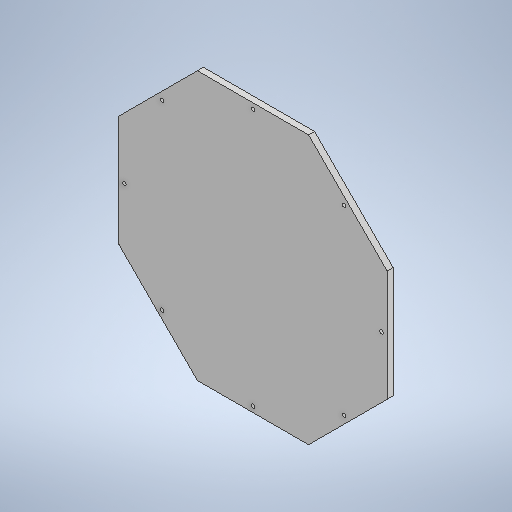
# Autodesk Inventor part: Cap
Saved by Autodesk Inventor 2025.1 (Build 291241020, 241B)
## iProperties
Created: 2024-09-21
Part Number: Cap
Material: 일반
Document SubType Name: Modeling
Designer: daare
Density: 1 g/cm^3
Appearance: 기본값
Author: daare
Autodesk Inventor part; units mm, degrees
ref_plane "YZ Plane" through (0, 0, 0) normal (1, 0, 0) x (0, 1, 0)
ref_plane "XZ Plane" through (0, 0, 0) normal (0, 1, 0) x (-1, 0, 0)
ref_plane "XY Plane" through (0, 0, 0) normal (0, 0, 1) x (1, 0, 0)
sketch "스케치1" plane through (0, 0, 0) normal (0, 0, 1) x (1, 0, 0)
  line L0 (112, -46.3919) -> (46.3919, -112)
  line L1 (46.3919, -112) -> (-46.3919, -112)
  line L2 (-46.3919, -112) -> (-112, -46.3919)
  line L3 (-112, -46.3919) -> (-112, 46.3919)
  line L4 (-112, 46.3919) -> (-46.3919, 112)
  line L5 (-46.3919, 112) -> (46.3919, 112)
  line L6 (46.3919, 112) -> (112, 46.3919)
  line L7 (112, 46.3919) -> (112, -46.3919)
  line L8 (0, 0) -> (-9.429, 0)
  line L9 (0, 0) -> (-9.429, 0)
  circle A0 centre (0, 107.302) radius 1.5
  circle A1 centre (-75.874, 75.874) radius 1.5
  circle A2 centre (-107.302, 0) radius 1.5
  circle A3 centre (-75.874, -75.874) radius 1.5
  circle A4 centre (0, -107.302) radius 1.5
  circle A5 centre (75.874, -75.874) radius 1.5
  circle A6 centre (107.302, 0) radius 1.5
  circle A7 centre (75.874, 75.874) radius 1.5
  dimension "d0" = 224
  dimension "d1" = 3
  dimension "d2" = 4.698
  dimension "d5" = 360
  constraints: 20 end point, 8 centre point, 2 horizontal, 1 coincident, 1 parallel, 1 vertical alignment, 34 other
  measures "d0" distance between parallel lines of L1 L5
  measures "d1" diameter of A0
  measures "d2" distance from line of L5 A0.centre
extrude "돌출1" add sketch "스케치1" along normal blind 5
